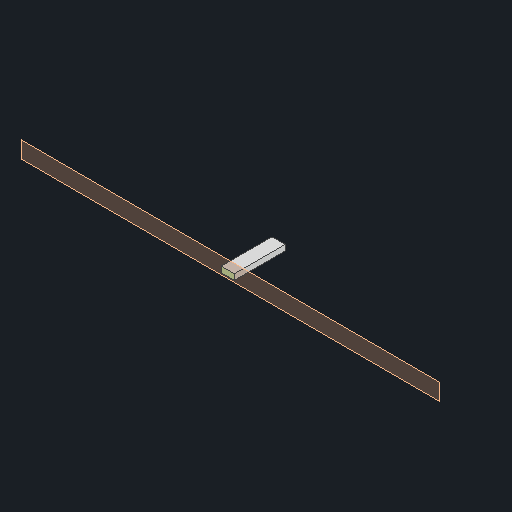
# Autodesk Inventor part: 2x4x13
Saved by Autodesk Inventor 2027 (Build 310192000, 192)
## iProperties
Created: 2026-08-07
Part Number: 2x4x13
Material: Generic
Document SubType Name: Modeling
Designer: lucas
Density: 1 g/cm^3
Appearance: Default
Author: lucas
Autodesk Inventor part; units mm, degrees
ref_plane "YZ Plane" through (0, 0, 0) normal (1, 0, 0) x (0, 1, 0)
ref_plane "XZ Plane" through (0, 0, 0) normal (0, 1, 0) x (-1, 0, 0)
ref_plane "XY Plane" through (0, 0, 0) normal (0, 0, 1) x (1, 0, 0)
ref_plane "Work Plane1" through (-1.616, 7.324, 0) normal (0, 0, 1) x (0.9999984, -0.0017691, 0)
sketch "Sketch1" plane through (-1.616, 7.324, 0) normal (0, 0, 1) x (0.9999984, -0.0017691, 0)
  line L0 (25.4962, -5.3592) -> (-63.4038, -5.3592)
  line L1 (-63.4038, -5.3592) -> (-63.4038, -43.4592)
  line L2 (-63.4038, -43.4592) -> (25.4962, -43.4592)
  line L3 (25.4962, -43.4592) -> (25.4962, -5.3592)
  point P0 (1.629, -7.3212)
  dimension "d2" = 88.9
  dimension "d3" = 38.1
  constraints: 8 end point, 2 parallel, 1 horizontal, 1 perpendicular
  measures "d2" distance of L1.end L2.end
  measures "d3" distance of L0.end L1.end
extrude "Extrusion1" add sketch "Sketch1" against normal blind 342.9
body "Solid1"
